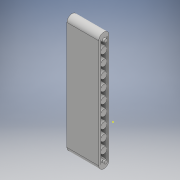
# Autodesk Inventor part: conveyer belt
Saved by Autodesk Inventor 2018 (Build 220112000, 112)
## iProperties
Created: 2018-01-21
Part Number: conveyer belt
Material: Generic
Document SubType Name: Modeling
Designer: Ahmed
Density: 1 g/cm^3
Appearance: Default
Author: Ahmed
Autodesk Inventor part; units mm, degrees
ref_plane "YZ Plane" through (0, 0, 0) normal (1, 0, 0) x (0, 1, 0)
ref_plane "XZ Plane" through (0, 0, 0) normal (0, 1, 0) x (-1, 0, 0)
ref_plane "XY Plane" through (0, 0, 0) normal (0, 0, 1) x (1, 0, 0)
sketch "Sketch1" plane through (0, 0, 0) normal (1, 0, 0) x (0, 1, 0)
  arc A0 (-194.1162, -481.5812) -> (-94.1162, -481.5812) centre (-144.1162, -481.5812) ccw
  line L0 (-194.1162, -481.5812) -> (-194.1162, 1218.4188)
  line L1 (-94.1162, 1218.4188) -> (-94.1162, -481.5812)
  arc A1 (-94.1162, 1218.4188) -> (-194.1162, 1218.4188) centre (-144.1162, 1218.4188) ccw
  line L2 (-64.1162, 1218.4188) -> (-64.1162, -481.5812)
  line L3 (-224.1162, 1218.4188) -> (-224.1162, -481.5812)
  arc A2 (-64.1162, 1218.4188) -> (-224.1162, 1218.4188) centre (-144.1162, 1218.4188) ccw
  arc A3 (-224.1162, -481.5812) -> (-64.1162, -481.5812) centre (-144.1162, -481.5812) ccw
  point P0 (0, 0)
  dimension "d5" = 1700
  dimension "d6" = 30
  dimension "d7" = 30
  constraints: 8 end point, 8 point on circle, 4 centre point, 2 coincident, 2 vertical, 1 parallel
  measures "d5" distance of L0.start L0.end
  measures "d6" distance between parallel lines of L0 L3
  measures "d7" distance between parallel lines of L1 L2
extrude "Extrusion1" add sketch "Sketch1" along normal mid plane 500 contours L0 A1 L1 A0 | L2 A3 L3 A2
sketch "Sketch2" plane through (250, 0, 0) normal (1, 0, 0) x (0, 0, -1)
  line L0 (-1218.4188, -94.1162) -> (481.5812, -94.1162)
  line L1 (481.5812, -194.1162) -> (-1218.4188, -194.1162)
  line L2 (481.5812, -64.1162) -> (-1218.4188, -64.1162) projected
  arc A0 (-1218.4188, -94.1162) -> (-1218.4188, -194.1162) centre (-1218.4188, -144.1162) ccw
  arc A1 (481.5812, -194.1162) -> (481.5812, -94.1162) centre (481.5812, -144.1162) ccw
  point P0 (0, 0)
  dimension "d10" = 1700
  dimension "d11" = 100
  dimension "d12" = 30
  constraints: 4 end point, 4 point on circle, 2 centre point, 1 horizontal, 1 parallel
  measures "d10" distance of L1.start L1.end
  measures "d11" distance of L0.end L1.start
  measures "d12" distance between parallel lines of L0 L2
extrude "Extrusion2" cut sketch "Sketch2" against normal blind 500
sketch "Sketch3" plane through (250, 0, 0) normal (1, 0, 0) x (0, 0, -1)
  circle A0 centre (-1048.4188, -144.1162) radius 50
  line L0 (-1218.4188, -94.1162) -> (481.5812, -94.1162) projected
  circle A1 centre (-878.4188, -144.1162) radius 50
  circle A2 centre (-708.4188, -144.1162) radius 50
  circle A3 centre (-538.4188, -144.1162) radius 50
  circle A4 centre (-368.4188, -144.1162) radius 50
  circle A5 centre (-198.4188, -144.1162) radius 50
  circle A6 centre (-28.4188, -144.1162) radius 50
  circle A7 centre (141.5812, -144.1162) radius 50
  circle A8 centre (311.5812, -144.1162) radius 50
  circle A9 centre (481.5812, -144.1162) radius 50
  circle A10 centre (-1218.4188, -144.1162) radius 50
  point P0 (0, 0)
  dimension "d17" = 170
  dimension "d18" = 170
  dimension "d19" = 170
  dimension "d20" = 170
  dimension "d21" = 170
  dimension "d23" = 170
  dimension "d24" = 170
  dimension "d25" = 170
  dimension "d26" = 170
  dimension "d27" = 170
  dimension "d28" = 0
  constraints: 11 centre point, 10 tangent
  measures "d17" distance of A9.centre A8.centre
  measures "d18" distance of A7.centre A8.centre
  measures "d19" distance of A6.centre A7.centre
  measures "d20" distance of A5.centre A6.centre
  measures "d21" distance of A5.centre A4.centre
  measures "d23" distance of A3.centre A4.centre
  measures "d24" distance of A3.centre A2.centre
  measures "d25" distance of A2.centre A1.centre
  measures "d26" distance of A1.centre A0.centre
  measures "d27" distance of A10.centre A0.centre
  measures "d28" horizontal distance of L0.start A10.centre
sketch "Sketch4" plane through (250, 0, 0) normal (1, 0, 0) x (0, 0, -1)
  point P0 (0, 0)
sketch "Sketch5" plane through (250, 0, 0) normal (1, 0, 0) x (0, 0, -1)
  point P0 (0, 0)
extrude "Extrusion3" add sketch "Sketch3" against normal blind 500
sketch "Sketch6" plane through (250, 0, 0) normal (1, 0, 0) x (0, 0, -1)
  circle A0 centre (-1193.419, -144.1162) radius 25
  circle A1 centre (456.581, -144.1162) radius 25
  point P0 (0, 0)
  dimension "d31" = 50
  dimension "d32" = 50
  constraints: 2 centre point
  measures "d31" diameter of A0
  measures "d32" diameter of A1
extrude "Extrusion4" add sketch "Sketch6" along normal blind 30 and the other way blind 530
body "Solid1"
